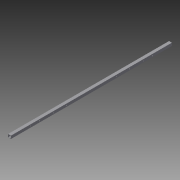
# Autodesk Inventor part: 1inSquareSupportOut
Saved by Autodesk Inventor 2016 (Build 200138000, 138)
## iProperties
Created: 2016-03-21
Part Number: 1inSquareSupportOut
Material: Generic
Document SubType Name: Modeling
Designer: Mac
Density: 1 g/cm^3
Appearance: Default
L2: 56.000 in
Author: Mac
Autodesk Inventor part; units mm, degrees
ref_plane "YZ Plane" through (0, 0, 0) normal (1, 0, 0) x (0, 1, 0)
ref_plane "XZ Plane" through (0, 0, 0) normal (0, 1, 0) x (-1, 0, 0)
ref_plane "XY Plane" through (0, 0, 0) normal (0, 0, 1) x (1, 0, 0)
sketch "Sketch1" plane through (0, 0, 0) normal (0, 0, 1) x (1, 0, 0)
  line L0 (-12.7, 12.7) -> (12.7, 12.7)
  line L1 (12.7, 12.7) -> (12.7, -12.7)
  line L2 (12.7, -12.7) -> (-12.7, -12.7)
  line L3 (-12.7, -12.7) -> (-12.7, 12.7)
  line L4 (9.652, 9.652) -> (-9.652, 9.652)
  line L5 (-9.652, 9.652) -> (-9.652, -9.652)
  line L6 (-9.652, -9.652) -> (9.652, -9.652)
  line L7 (9.652, -9.652) -> (9.652, 9.652)
  point P0 (0, 0)
  point P1 (12.7, 0)
  point P2 (0, 12.7)
  dimension "d0" = 25.4
  dimension "d1" = 25.4
  dimension "d2" = 3.048
  constraints: 16 end point, 4 parallel, 2 midpoint, 2 perpendicular, 1 horizontal, 1 horizontal alignment, 1 vertical alignment, 3 other
  measures "d0" distance of L0.start L0.end
  measures "d1" distance of L0.end L1.end
  measures "d2" distance between parallel lines of L4 L0
extrude "Extrusion1" add sketch "Sketch1" along normal mid plane 1422.4
sketch "Sketch2" plane through (0, 0, 0) normal (0, 0, 1) x (1, 0, 0)
  point P0 (0, 0)
sketch "Sketch3" plane through (12.7, 12.7, 711.2) normal (1, 0, 0) x (0, 0, -1)
  circle A0 centre (1248.4758, -12.693) radius 4.25 projected
  circle A1 centre (1168.4758, -12.693) radius 4.4 projected
  circle A2 centre (253.9242, -12.693) radius 4.4 projected
  circle A3 centre (173.9242, -12.693) radius 4.25 projected
  point P0 (711.2, -12.7)
  point P1 (488.8742, -12.693)
  point P2 (374.5742, -12.693)
  point P3 (933.5258, -12.693)
  point P4 (1047.8258, -12.693)
  dimension "d5" = 114.3
  dimension "d6" = 120.65
  dimension "d7" = 120.65
  dimension "d8" = 114.3
  constraints: 5 horizontal alignment, 4 coincident
  measures "d5" distance of point (488.874, -12.693) point (374.574, -12.693)
  measures "d6" distance of point (253.924, -12.693) point (374.574, -12.693)
  measures "d7" distance of point (1047.826, -12.693) point (1168.476, -12.693)
  measures "d8" distance of point (933.526, -12.693) point (1047.826, -12.693)
hole "Hole1" at (12.7, 0.007, -537.2758) at (12.7, 0.007, -457.2758) at (12.7, 0.007, -336.6258) at (12.7, 0.007, -222.3258) at (12.7, 0.007, 222.3258) at (12.7, 0.007, 336.6258) at (12.7, 0.007, 457.2758) at (12.7, 0.007, 537.2758) direction (-1, 0, 0) diameter 6.7469 depth 3.175 tip angle 118
sketch "Sketch4" plane through (-12.7, -12.7, -711.2) normal (-1, 0, 0) x (0, 0, 1)
  circle A0 centre (173.9242, 12.707) radius 3.3734 projected
  circle A1 centre (253.9242, 12.707) radius 3.3734 projected
  circle A2 centre (374.5742, 12.707) radius 3.3734 projected
  circle A3 centre (488.8742, 12.707) radius 3.3734 projected
  circle A4 centre (933.5258, 12.707) radius 3.3734 projected
  circle A5 centre (1047.8258, 12.707) radius 3.3734 projected
  circle A6 centre (1168.4758, 12.707) radius 3.3734 projected
  circle A7 centre (1248.4758, 12.707) radius 3.3734 projected
  point P0 (711.2, 12.7)
  constraints: 8 coincident
hole "Hole2" at (-12.7, 0.007, 537.2758) at (-12.7, 0.007, 457.2758) at (-12.7, 0.007, 336.6258) at (-12.7, 0.007, 222.3258) at (-12.7, 0.007, -222.3258) at (-12.7, 0.007, -336.6258) at (-12.7, 0.007, -457.2758) at (-12.7, 0.007, -537.2758) direction (1, 0, 0) diameter 12.7 depth 3.175 tip angle 118
equation "\"d2\" = thick"
equation "\"d3\" = L2"
equation "\"L\" = 1219.2"
equation "\"thick\" = 3.048"
equation "\"L2\" = 1422.4"
body "Solid1"
